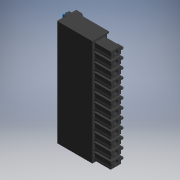
# Autodesk Inventor part: 3943083 12GD-1RR3,5-CLP-CBL
Saved by Autodesk Inventor 2017.3 (Build 213256000, 256)
## iProperties
Part Number: 3943083 12GD-1RR3,5-CLP-CBL
Material: Generic
Catalog Web Link: www.cadenas.de
Description: NEKM-C6 (p)-Terminal strip
Vendor: FESTO
Document SubType Name: Modeling
Designer: partserver
Manufacturer: FESTO
Mass: 4.97851 g
Surface Area: 43.3437 cm^2
Volume: 4.97851 cm^3
Density: 1 g/cm^3
Appearance: PSOLRGB-80-80-80
Category: PARTsolutions
Company: FESTO
Title: 3943083 12GD-1RR3,5-CLP-CBL
Author: Cadenas PARTsolutions
Comments: Terminal strip
PSOL_IDENT_0: {$CADENAS_DATA\23d-libs\festo\parts\n\nekm\parts\nekm_c6_parts.prj},199 {VTYP=3D},{NB=3943083 12GD-1
PSOL_IDENT_1: RR3,5-CLP-CBL},{LINA=3943083 12GD-1RR3,5-CLP-CBL},{NN=NEKM-C6 (p)},{DATE=16.05.2019 05:36:58},{GEOMD
PSOL_IDENT_2: ATE=16.05.2019 05:36:56},{VERSION=},{LINEID=50},{WBVAR=},{WBNUMERIC=}  {NB=3943083 12GD-1RR3,5-CLP-C
PSOL_IDENT_3: BL},{LINA=3943083 12GD-1RR3,5-CLP-CBL},{KT=DUMMY},{TNR=3943083},{TYP=12GD-1RR3,5-CLP-CBL},{VERS=3},{
PSOL_IDENT_4: N=12},{L=42.750},{L1=0.000}
NB: 3943083 12GD-1RR3,5-CLP-CBL
NN: NEKM-C6 (p)
NT: Terminal strip
NBSYN: $TNR. $TYP.
LINA: 3943083 12GD-1RR3,5-CLP-CBL
CATALOG: Festo
TNR: 3943083
TYP: 12GD-1RR3,5-CLP-CBL
VERS: 3
N: 12
L: 42.75
L1: 0
SUPPLIER: FESTO
ARTICLENO: 3943083 12GD-1RR3,5-CLP-CBL
BOMINFO: 3943083 12GD-1RR3,5-CLP-CBL
CREATOR: CADENAS GmbH
Autodesk Inventor part; units mm, degrees
sketch "Sketch_1" plane through (0, 0, 0) normal (0, 0, 1) x (1, 0, 0)
  line L0 (0, 2.675) -> (0, -3.875)
  line L1 (0, -3.875) -> (14.1, -3.875)
  arc A0 (14.1, -3.875) -> (14.3, -3.675) centre (14.1, -3.675) ccw
  line L2 (14.3, -3.675) -> (14.3, 3.675)
  arc A1 (14.3, 3.675) -> (14.1, 3.875) centre (14.1, 3.675) ccw
  line L3 (14.1, 3.875) -> (12, 3.875)
  line L4 (12, 3.875) -> (10.4412, 2.975)
  line L5 (10.4412, 2.975) -> (0.3, 2.975)
  arc A2 (0.3, 2.975) -> (0, 2.675) centre (0.3, 2.675) ccw
  constraints: 12 end point, 6 point on circle, 3 centre point
extrude "Extrusion1" add sketch "Sketch_1" along normal mid plane 42.75
sketch "Sketch_2" plane through (0, 0, 0) normal (0, 0, 1) x (1, 0, 0)
  line L0 (0, 1.025) -> (0.6, 1.025)
  arc A0 (0.6, 1.025) -> (0.9, 1.325) centre (0.6, 1.325) ccw
  line L1 (0.9, 1.325) -> (0.9, 2.975)
  line L2 (0.9, 2.975) -> (0, 2.975)
  line L3 (0, 2.975) -> (0, 1.025)
  constraints: 8 end point, 2 point on circle, 1 centre point
extrude "Extrusion2" cut sketch "Sketch_2" along normal mid plane 41.85
sketch "Sketch_3" plane through (0, 0, 21.375) normal (0, 0, 1) x (1, 0, 0)
  line L0 (14.3, 2.225) -> (14.3, -0.5681)
  arc A0 (14.4, -0.3949) -> (14.3, -0.5681) centre (14.5, -0.5681) ccw
  line L1 (14.4, -0.3949) -> (15.2, 0.067)
  arc A1 (15.2, 0.067) -> (15.3, 0.2402) centre (15.1, 0.2402) ccw
  line L2 (15.3, 0.2402) -> (15.3, 1.825)
  arc A2 (15.3, 1.825) -> (15.1, 2.025) centre (15.1, 1.825) ccw
  line L3 (15.1, 2.025) -> (14.5, 2.025)
  arc A3 (14.3, 2.225) -> (14.5, 2.025) centre (14.5, 2.225) ccw
  constraints: 8 end point, 8 point on circle, 4 centre point
extrude "Extrusion3" add sketch "Sketch_3" against normal blind 0.6
sketch "Sketch_4" plane through (0, 0, -21.375) normal (0, 0, 1) x (1, 0, 0)
  line L0 (14.3, 2.225) -> (14.3, -0.5681)
  arc A0 (14.4, -0.3949) -> (14.3, -0.5681) centre (14.5, -0.5681) ccw
  line L1 (14.4, -0.3949) -> (15.2, 0.067)
  arc A1 (15.2, 0.067) -> (15.3, 0.2402) centre (15.1, 0.2402) ccw
  line L2 (15.3, 0.2402) -> (15.3, 1.825)
  arc A2 (15.3, 1.825) -> (15.1, 2.025) centre (15.1, 1.825) ccw
  line L3 (15.1, 2.025) -> (14.5, 2.025)
  arc A3 (14.3, 2.225) -> (14.5, 2.025) centre (14.5, 2.225) ccw
  constraints: 8 end point, 8 point on circle, 4 centre point
extrude "Extrusion4" add sketch "Sketch_4" along normal blind 0.6
sketch "Sketch_5" plane through (0, 0, 17.725) normal (0, 0, 1) x (1, 0, 0)
  line L0 (14.3, 2.225) -> (14.3, -0.5681)
  arc A0 (14.4, -0.3949) -> (14.3, -0.5681) centre (14.5, -0.5681) ccw
  line L1 (14.4, -0.3949) -> (15.2, 0.067)
  arc A1 (15.2, 0.067) -> (15.3, 0.2402) centre (15.1, 0.2402) ccw
  line L2 (15.3, 0.2402) -> (15.3, 1.825)
  arc A2 (15.3, 1.825) -> (15.1, 2.025) centre (15.1, 1.825) ccw
  line L3 (15.1, 2.025) -> (14.5, 2.025)
  arc A3 (14.3, 2.225) -> (14.5, 2.025) centre (14.5, 2.225) ccw
  constraints: 8 end point, 8 point on circle, 4 centre point
extrude "Extrusion5" add sketch "Sketch_5" against normal blind 0.45
pattern_linear "Rectangular Pattern1" count 11 spacing 3.5 along (0, 0, -1) of "Extrusion5"
sketch "Sketch_7" plane through (0, 0, 20.675) normal (0, 0, 1) x (1, 0, 0)
  line L0 (14.3, 0.225) -> (16.1, 0.225)
  arc A0 (16.1, 0.225) -> (16.3, 0.425) centre (16.1, 0.425) ccw
  line L1 (16.3, 0.425) -> (16.3, 0.4497)
  arc A1 (16.3, 0.4497) -> (16.1261, 0.648) centre (16.1, 0.4497) ccw
  line L2 (16.1261, 0.648) -> (15.1418, 0.7776)
  arc A2 (15.1418, 1.3724) -> (15.1418, 0.7776) centre (15.181, 1.075) ccw
  line L3 (15.1418, 1.3724) -> (16.1261, 1.502)
  arc A3 (16.1261, 1.502) -> (16.3, 1.7003) centre (16.1, 1.7003) ccw
  line L4 (16.3, 1.7003) -> (16.3, 1.725)
  arc A4 (16.3, 1.725) -> (16.1, 1.925) centre (16.1, 1.725) ccw
  line L5 (16.1, 1.925) -> (14.3, 1.925)
  line L6 (14.3, 1.925) -> (14.3, 0.225)
  constraints: 14 end point, 10 point on circle, 5 centre point
extrude "Extrusion6" add sketch "Sketch_7" against normal blind 2.85
pattern_linear "Rectangular Pattern2" count 12 spacing 3.5 along (0, 0, -1) of "Extrusion6"
sketch "Sketch_9" plane through (0, -1.825, 0) normal (0, 1, 0) x (1, 0, 0)
  line L0 (14.3, -19.375) -> (11.3, -19.375)
  line L1 (11.3, -19.375) -> (11.3, -17.875)
  line L2 (11.3, -17.875) -> (14.1, -17.875)
  arc A0 (14.1, -17.875) -> (14.3, -17.675) centre (14.1, -17.675) ccw
  line L3 (14.3, -17.675) -> (14.3, -19.375)
  line L4 (14.3, -19.375) -> (11.3, -19.375)
  constraints: 10 end point, 2 point on circle, 1 centre point
revolve "Revolution1" cut sketch "Sketch_9" angle 360 about axis through (14.3, -1.825, 19.375) along (1, 0, 0)
pattern_linear "Rectangular Pattern3" count 12 spacing 3.5 along (0, 0, -1) of "Revolution1"
sketch "Sketch_12" plane through (4.9, 0, 0) normal (1, 0, 0) x (0, 0, -1)
  line L0 (-20.875, 2.975) -> (-17.625, 2.975)
  arc A0 (-17.625, 2.975) -> (-18.525, 3.875) centre (-18.525, 2.975) ccw
  line L1 (-18.525, 3.875) -> (-19.975, 3.875)
  arc A1 (-19.975, 3.875) -> (-20.875, 2.975) centre (-19.975, 2.975) ccw
  constraints: 4 end point, 4 point on circle, 2 centre point
extrude "Extrusion7" add sketch "Sketch_12" along normal blind 8
pattern_linear "Rectangular Pattern4" count 12 spacing 3.5 along (0, 0, -1) of "Extrusion7"
sketch "Sketch_14" plane through (0, 0, 0) normal (0, 0, 1) x (1, 0, 0)
  line L0 (2, 3.875) -> (2, 2.975)
  line L1 (2, 2.975) -> (4.9, 2.975)
  line L2 (4.9, 2.975) -> (6.4588, 3.875)
  line L3 (6.4588, 3.875) -> (2, 3.875)
  constraints: 8 end point
extrude "Extrusion8" cut sketch "Sketch_14" along normal mid plane 42.75
sketch "Sketch_11" plane through (14.3, 0, 0) normal (1, 0, 0) x (0, 0, -1)
  line L0 (-20.275, 2.974) -> (-20.275, 1.925)
  line L1 (-20.275, 1.925) -> (-18.225, 1.925)
  line L2 (-18.225, 1.925) -> (-18.225, 2.974)
  arc A0 (-18.225, 2.974) -> (-18.526, 3.275) centre (-18.526, 2.974) ccw
  line L3 (-18.526, 3.275) -> (-19.974, 3.275)
  arc A1 (-19.974, 3.275) -> (-20.275, 2.974) centre (-19.974, 2.974) ccw
  constraints: 8 end point, 4 point on circle, 2 centre point
extrude "Extrusion9" cut sketch "Sketch_11" against normal blind 4
pattern_linear "Rectangular Pattern5" count 12 spacing 3.5 along (0, 0, -1) of "Extrusion9"
sketch "Sketch_16" plane through (0, 0, 0) normal (1, 0, 0) x (0, 1, 0)
  line L0 (-3.075, 20.625) -> (-3.075, 20.1987)
  arc A0 (-3.075, 18.3013) -> (-3.075, 20.1987) centre (-4.425, 19.25) ccw
  line L1 (-3.075, 18.3013) -> (-3.075, 17.875)
  line L2 (-3.075, 17.875) -> (1.025, 17.875)
  line L3 (1.025, 17.875) -> (1.025, 20.625)
  line L4 (1.025, 20.625) -> (-3.075, 20.625)
  constraints: 10 end point, 2 point on circle, 1 centre point
extrude "Extrusion10" add sketch "Sketch_16" against normal blind 6.6
pattern_linear "Rectangular Pattern6" count 12 spacing 3.5 along (0, 0, -1) of "Extrusion10"
sketch "Sketch_18" plane through (0, -0.875, 0) normal (0, 1, 0) x (1, 0, 0)
  line L0 (-5.6, -19.25) -> (-6.6, -19.25)
  line L1 (-6.6, -19.25) -> (-6.6, -18.45)
  line L2 (-6.6, -18.45) -> (-5.6, -18.45)
  line L3 (-5.6, -18.45) -> (-5.6, -19.25)
  line L4 (-5.6, -19.25) -> (-6.6, -19.25)
  constraints: 10 end point
revolve "Revolution2" cut sketch "Sketch_18" angle 360 about axis through (-5.6, -0.875, 19.25) along (1, 0, 0)
pattern_linear "Rectangular Pattern7" count 12 spacing 3.5 along (0, 0, -1) of "Revolution2"
sketch "Sketch_20" plane through (-6.35, 0, 0) normal (1, 0, 0) x (0, 0, -1)
  line L0 (-19.65, 2.125) -> (-19.65, 1.025)
  line L1 (-19.65, 1.025) -> (-18.85, 1.025)
  line L2 (-18.85, 1.025) -> (-18.85, 2.125)
  arc A0 (-18.85, 2.125) -> (-19.05, 2.325) centre (-19.05, 2.125) ccw
  line L3 (-19.05, 2.325) -> (-19.45, 2.325)
  arc A1 (-19.45, 2.325) -> (-19.65, 2.125) centre (-19.45, 2.125) ccw
  constraints: 8 end point, 4 point on circle, 2 centre point
extrude "Extrusion11" add sketch "Sketch_20" along normal blind 2.25
pattern_linear "Rectangular Pattern8" count 12 spacing 3.5 along (0, 0, -1) of "Extrusion11"
ref_plane "ANBAU_XY" through (0, 0, 0) normal (0, 1, 0) x (1, 0, 0)
ref_plane "ANBAU_YZ" through (0, 0, 0) normal (1, 0, 0) x (0, 0, -1)
ref_plane "ANBAU_ZX" through (0, 0, 0) normal (0, 0, -1) x (0, 1, 0)
body "Solid1"
